Autodesk Inventor part; units mm, degrees
(part 2 of 2)
  line L765 (55.2108, -84.3874) -> (55.2873, -85.0207)
  line L766 (55.2873, -85.0207) -> (55.3337, -85.6628)
  line L767 (55.3337, -85.6628) -> (55.3494, -86.313)
  line L768 (75.3327, -73.346) -> (75.3327, -77.0507)
  line L769 (75.3327, -77.0507) -> (60.5124, -77.0507)
  line L770 (60.5124, -77.0507) -> (60.5124, -73.346)
  line L771 (60.5124, -73.346) -> (75.3327, -73.346)
  line L772 (60.513, -84.5139) -> (73.48, -84.5139)
  line L773 (73.48, -84.5139) -> (73.48, -88.1663)
  line L774 (73.48, -88.1663) -> (64.2178, -88.1663)
  line L775 (64.2178, -88.1663) -> (64.2178, -99.2813)
  line L776 (64.2178, -99.2813) -> (60.513, -99.2813)
  line L777 (60.513, -99.2813) -> (60.513, -84.5139)
  line L778 (79.5669, -73.346) -> (96.8562, -73.346)
  line L779 (96.8562, -73.346) -> (96.8562, -76.9851)
  line L780 (96.8562, -76.9851) -> (79.5669, -76.9851)
  line L781 (79.5669, -76.9851) -> (79.5669, -73.346)
  line L782 (86.3592, -99.2807) -> (86.3592, -79.0998)
  line L783 (86.3592, -79.0998) -> (90.064, -79.0998)
  line L784 (90.064, -79.0998) -> (90.064, -99.2813)
  line L785 (90.064, -99.2813) -> (86.3592, -99.2813)
  line L786 (86.3592, -99.2813) -> (86.3592, -99.2807)
  line L787 (108.9957, -95.7819) -> (108.9957, -99.5463)
  line L788 (108.9957, -99.5463) -> (108.5376, -99.5)
  line L789 (108.5376, -99.5) -> (108.0916, -99.4372)
  line L790 (108.0916, -99.4372) -> (107.6576, -99.3582)
  line L791 (107.6576, -99.3582) -> (107.2359, -99.2632)
  line L792 (107.2359, -99.2632) -> (106.8264, -99.1526)
  line L793 (106.8264, -99.1526) -> (106.4293, -99.0265)
  line L794 (106.4293, -99.0265) -> (106.0448, -98.8854)
  line L795 (106.0448, -98.8854) -> (105.6728, -98.7294)
  line L796 (105.6728, -98.7294) -> (105.3136, -98.5588)
  line L797 (105.3136, -98.5588) -> (104.9672, -98.374)
  line L798 (104.9672, -98.374) -> (104.6337, -98.1751)
  line L799 (104.6337, -98.1751) -> (104.3132, -97.9625)
  line L800 (104.3132, -97.9625) -> (104.0059, -97.7364)
  line L801 (104.0059, -97.7364) -> (103.7118, -97.4972)
  line L802 (103.7118, -97.4972) -> (103.431, -97.245)
  line L803 (103.431, -97.245) -> (103.1637, -96.9803)
  line L804 (103.1637, -96.9803) -> (102.9099, -96.7031)
  line L805 (102.9099, -96.7031) -> (102.6698, -96.4139)
  line L806 (102.6698, -96.4139) -> (102.4434, -96.1129)
  line L807 (102.4434, -96.1129) -> (102.2309, -95.8004)
  line L808 (102.2309, -95.8004) -> (102.0324, -95.4767)
  line L809 (102.0324, -95.4767) -> (101.8479, -95.1419)
  line L810 (101.8479, -95.1419) -> (101.6776, -94.7965)
  line L811 (101.6776, -94.7965) -> (101.5216, -94.4407)
  line L812 (101.5216, -94.4407) -> (101.38, -94.0748)
  line L813 (101.38, -94.0748) -> (101.2528, -93.6989)
  line L814 (101.2528, -93.6989) -> (101.1403, -93.3135)
  line L815 (101.1403, -93.3135) -> (101.0424, -92.9188)
  line L816 (101.0424, -92.9188) -> (100.9594, -92.5151)
  line L817 (100.9594, -92.5151) -> (100.8912, -92.1026)
  line L818 (100.8912, -92.1026) -> (100.8381, -91.6817)
  line L819 (100.8381, -91.6817) -> (100.8001, -91.2525)
  line L820 (100.8001, -91.2525) -> (104.5012, -90.6352)
  line L821 (104.5012, -90.6352) -> (104.5694, -91.1029)
  line L822 (104.5694, -91.1029) -> (104.6601, -91.56)
  line L823 (104.6601, -91.56) -> (104.7745, -92.0048)
  line L824 (104.7745, -92.0048) -> (104.9139, -92.4353)
  line L825 (104.9139, -92.4353) -> (105.0796, -92.8494)
  line L826 (105.0796, -92.8494) -> (105.2728, -93.2454)
  line L827 (105.2728, -93.2454) -> (105.4947, -93.6213)
  line L828 (105.4947, -93.6213) -> (105.7467, -93.9752)
  line L829 (105.7467, -93.9752) -> (106.0301, -94.3051)
  line L830 (106.0301, -94.3051) -> (106.3459, -94.6092)
  line L831 (106.3459, -94.6092) -> (106.6956, -94.8854)
  line L832 (106.6956, -94.8854) -> (107.0804, -95.1319)
  line L833 (107.0804, -95.1319) -> (107.2864, -95.2435)
  line L834 (107.2864, -95.2435) -> (107.5016, -95.3468)
  line L835 (107.5016, -95.3468) -> (107.7262, -95.4418)
  line L836 (107.7262, -95.4418) -> (107.9603, -95.5282)
  line L837 (107.9603, -95.5282) -> (108.2042, -95.6057)
  line L838 (108.2042, -95.6057) -> (108.4579, -95.674)
  line L839 (108.4579, -95.674) -> (108.7217, -95.7331)
  line L840 (108.7217, -95.7331) -> (108.9957, -95.7825)
  line L841 (108.9957, -95.7825) -> (108.9957, -95.7819)
  line L842 (108.9957, -73.0972) -> (108.9957, -76.8448)
  line L843 (108.9957, -76.8448) -> (108.7303, -76.8953)
  line L844 (108.7303, -76.8953) -> (108.4771, -76.9554)
  line L845 (108.4771, -76.9554) -> (108.2356, -77.0248)
  line L846 (108.2356, -77.0248) -> (108.0057, -77.1031)
  line L847 (108.0057, -77.1031) -> (107.787, -77.1901)
  line L848 (107.787, -77.1901) -> (107.5792, -77.2854)
  line L849 (107.5792, -77.2854) -> (107.3821, -77.3887)
  line L850 (107.3821, -77.3887) -> (107.1954, -77.4997)
  line L851 (107.1954, -77.4997) -> (107.0188, -77.6182)
  line L852 (107.0188, -77.6182) -> (106.8519, -77.7437)
  line L853 (106.8519, -77.7437) -> (106.5465, -78.0148)
  line L854 (106.5465, -78.0148) -> (106.2768, -78.3107)
  line L855 (106.2768, -78.3107) -> (106.0406, -78.6288)
  line L856 (106.0406, -78.6288) -> (105.8355, -78.9667)
  line L857 (105.8355, -78.9667) -> (105.6593, -79.3219)
  line L858 (105.6593, -79.3219) -> (105.5096, -79.692)
  line L859 (105.5096, -79.692) -> (105.3842, -80.0745)
  line L860 (105.3842, -80.0745) -> (105.2808, -80.467)
  line L861 (105.2808, -80.467) -> (105.1971, -80.8669)
  line L862 (105.1971, -80.8669) -> (105.1307, -81.2719)
  line L863 (105.1307, -81.2719) -> (105.0795, -81.6795)
  line L864 (105.0795, -81.6795) -> (101.3783, -81.0621)
  line L865 (101.3783, -81.0621) -> (101.4195, -80.6638)
  line L866 (101.4195, -80.6638) -> (101.4761, -80.272)
  line L867 (101.4761, -80.272) -> (101.5478, -79.8871)
  line L868 (101.5478, -79.8871) -> (101.6343, -79.5093)
  line L869 (101.6343, -79.5093) -> (101.7355, -79.139)
  line L870 (101.7355, -79.139) -> (101.8509, -78.7765)
  line L871 (101.8509, -78.7765) -> (101.9804, -78.422)
  line L872 (101.9804, -78.422) -> (102.1237, -78.076)
  line L873 (102.1237, -78.076) -> (102.2804, -77.7387)
  line L874 (102.2804, -77.7387) -> (102.4504, -77.4103)
  line L875 (102.4504, -77.4103) -> (102.6334, -77.0913)
  line L876 (102.6334, -77.0913) -> (102.829, -76.782)
  line L877 (102.829, -76.782) -> (103.0371, -76.4826)
  line L878 (103.0371, -76.4826) -> (103.2573, -76.1934)
  line L879 (103.2573, -76.1934) -> (103.4895, -75.9148)
  line L880 (103.4895, -75.9148) -> (103.7332, -75.6471)
  line L881 (103.7332, -75.6471) -> (103.9883, -75.3906)
  line L882 (103.9883, -75.3906) -> (104.2545, -75.1456)
  line L883 (104.2545, -75.1456) -> (104.5316, -74.9124)
  line L884 (104.5316, -74.9124) -> (104.8191, -74.6913)
  line L885 (104.8191, -74.6913) -> (105.117, -74.4827)
  line L886 (105.117, -74.4827) -> (105.4248, -74.2868)
  line L887 (105.4248, -74.2868) -> (105.7425, -74.1039)
  line L888 (105.7425, -74.1039) -> (106.0695, -73.9344)
  line L889 (106.0695, -73.9344) -> (106.4058, -73.7786)
  line L890 (106.4058, -73.7786) -> (106.751, -73.6367)
  line L891 (106.751, -73.6367) -> (107.1049, -73.5092)
  line L892 (107.1049, -73.5092) -> (107.4672, -73.3962)
  line L893 (107.4672, -73.3962) -> (107.8377, -73.2982)
  line L894 (107.8377, -73.2982) -> (108.216, -73.2153)
  line L895 (108.216, -73.2153) -> (108.6018, -73.148)
  line L896 (108.6018, -73.148) -> (108.9951, -73.0966)
  line L897 (108.9951, -73.0966) -> (108.9957, -73.0972)
  line L898 (119.306, -91.2525) -> (119.2993, -91.5962)
  line L899 (119.2993, -91.5962) -> (119.2793, -91.9424)
  line L900 (119.2793, -91.9424) -> (119.2455, -92.2901)
  line L901 (119.2455, -92.2901) -> (119.1978, -92.6387)
  line L902 (119.1978, -92.6387) -> (119.1358, -92.9874)
  line L903 (119.1358, -92.9874) -> (119.0594, -93.3353)
  line L904 (119.0594, -93.3353) -> (118.9681, -93.6817)
  line L905 (118.9681, -93.6817) -> (118.8619, -94.0258)
  line L906 (118.8619, -94.0258) -> (118.7403, -94.3667)
  line L907 (118.7403, -94.3667) -> (118.6032, -94.7039)
  line L908 (118.6032, -94.7039) -> (118.4503, -95.0363)
  line L909 (118.4503, -95.0363) -> (118.2812, -95.3633)
  line L910 (118.2812, -95.3633) -> (118.0958, -95.684)
  line L911 (118.0958, -95.684) -> (117.8938, -95.9977)
  line L912 (117.8938, -95.9977) -> (117.6749, -96.3036)
  line L913 (117.6749, -96.3036) -> (117.4388, -96.6009)
  line L914 (117.4388, -96.6009) -> (117.1853, -96.8889)
  line L915 (117.1853, -96.8889) -> (116.9141, -97.1666)
  line L916 (116.9141, -97.1666) -> (116.6249, -97.4334)
  line L917 (116.6249, -97.4334) -> (116.3175, -97.6884)
  line L918 (116.3175, -97.6884) -> (115.9917, -97.9309)
  line L919 (115.9917, -97.9309) -> (115.647, -98.16)
  line L920 (115.647, -98.16) -> (115.2834, -98.3751)
  line L921 (115.2834, -98.3751) -> (114.9004, -98.5752)
  line L922 (114.9004, -98.5752) -> (114.4979, -98.7597)
  line L923 (114.4979, -98.7597) -> (114.0756, -98.9277)
  line L924 (114.0756, -98.9277) -> (113.6331, -99.0784)
  line L925 (113.6331, -99.0784) -> (113.1704, -99.2111)
  line L926 (113.1704, -99.2111) -> (112.687, -99.325)
  line L927 (112.687, -99.325) -> (112.1827, -99.4192)
  line L928 (112.1827, -99.4192) -> (111.6572, -99.4931)
  line L929 (111.6572, -99.4931) -> (111.1104, -99.5457)
  line L930 (111.1104, -99.5457) -> (111.1104, -95.8234)
  line L931 (111.1104, -95.8234) -> (111.6337, -95.7501)
  line L932 (111.6337, -95.7501) -> (112.1273, -95.643)
  line L933 (112.1273, -95.643) -> (112.5907, -95.5038)
  line L934 (112.5907, -95.5038) -> (113.0232, -95.3344)
  line L935 (113.0232, -95.3344) -> (113.4244, -95.1363)
  line L936 (113.4244, -95.1363) -> (113.7936, -94.9114)
  line L937 (113.7936, -94.9114) -> (114.1303, -94.6612)
  line L938 (114.1303, -94.6612) -> (114.4339, -94.3877)
  line L939 (114.4339, -94.3877) -> (114.7039, -94.0924)
  line L940 (114.7039, -94.0924) -> (114.9397, -93.7771)
  line L941 (114.9397, -93.7771) -> (115.1408, -93.4436)
  line L942 (115.1408, -93.4436) -> (115.3065, -93.0934)
  line L943 (115.3065, -93.0934) -> (115.4364, -92.7284)
  line L944 (115.4364, -92.7284) -> (115.5299, -92.3503)
  line L945 (115.5299, -92.3503) -> (115.5864, -91.9608)
  line L946 (115.5864, -91.9608) -> (115.6054, -91.5615)
  line L947 (115.6054, -91.5615) -> (115.5845, -91.1111)
  line L948 (115.5845, -91.1111) -> (115.5227, -90.6978)
  line L949 (115.5227, -90.6978) -> (115.4769, -90.5047)
  line L950 (115.4769, -90.5047) -> (115.4214, -90.3202)
  line L951 (115.4214, -90.3202) -> (115.3564, -90.1443)
  line L952 (115.3564, -90.1443) -> (115.2819, -89.9768)
  line L953 (115.2819, -89.9768) -> (115.1982, -89.8174)
  line L954 (115.1982, -89.8174) -> (115.1055, -89.6659)
  line L955 (115.1055, -89.6659) -> (115.0038, -89.5222)
  line L956 (115.0038, -89.5222) -> (114.8935, -89.3861)
  line L957 (114.8935, -89.3861) -> (114.6473, -89.1357)
  line L958 (114.6473, -89.1357) -> (114.3682, -88.9133)
  line L959 (114.3682, -88.9133) -> (114.0575, -88.7174)
  line L960 (114.0575, -88.7174) -> (113.7166, -88.5462)
  line L961 (113.7166, -88.5462) -> (113.3467, -88.3985)
  line L962 (113.3467, -88.3985) -> (112.9493, -88.2725)
  line L963 (112.9493, -88.2725) -> (112.5256, -88.1667)
  line L964 (112.5256, -88.1667) -> (112.077, -88.0797)
  line L965 (112.077, -88.0797) -> (111.6048, -88.0098)
  line L966 (111.6048, -88.0098) -> (111.1104, -87.9555)
  line L967 (111.1104, -87.9555) -> (111.1104, -83.9201)
  line L968 (111.1104, -83.9201) -> (111.4723, -83.8432)
  line L969 (111.4723, -83.8432) -> (111.8318, -83.7523)
  line L970 (111.8318, -83.7523) -> (112.1858, -83.6464)
  line L971 (112.1858, -83.6464) -> (112.5315, -83.5245)
  line L972 (112.5315, -83.5245) -> (112.866, -83.3856)
  line L973 (112.866, -83.3856) -> (113.1866, -83.2287)
  line L974 (113.1866, -83.2287) -> (113.4902, -83.0527)
  line L975 (113.4902, -83.0527) -> (113.7741, -82.8567)
  line L976 (113.7741, -82.8567) -> (114.0353, -82.6396)
  line L977 (114.0353, -82.6396) -> (114.271, -82.4004)
  line L978 (114.271, -82.4004) -> (114.4783, -82.1382)
  line L979 (114.4783, -82.1382) -> (114.6544, -81.8519)
  line L980 (114.6544, -81.8519) -> (114.7963, -81.5404)
  line L981 (114.7963, -81.5404) -> (114.9012, -81.2029)
  line L982 (114.9012, -81.2029) -> (114.9389, -81.024)
  line L983 (114.9389, -81.024) -> (114.9663, -80.8382)
  line L984 (114.9663, -80.8382) -> (114.983, -80.6453)
  line L985 (114.983, -80.6453) -> (114.9886, -80.4453)
  line L986 (114.9886, -80.4453) -> (114.9742, -80.1536)
  line L987 (114.9742, -80.1536) -> (114.9307, -79.8588)
  line L988 (114.9307, -79.8588) -> (114.858, -79.5634)
  line L989 (114.858, -79.5634) -> (114.7556, -79.2699)
  line L990 (114.7556, -79.2699) -> (114.6233, -78.9808)
  line L991 (114.6233, -78.9808) -> (114.4608, -78.6986)
  line L992 (114.4608, -78.6986) -> (114.2678, -78.4258)
  line L993 (114.2678, -78.4258) -> (114.044, -78.1649)
  line L994 (114.044, -78.1649) -> (113.7891, -77.9184)
  line L995 (113.7891, -77.9184) -> (113.5029, -77.6888)
  line L996 (113.5029, -77.6888) -> (113.185, -77.4786)
  line L997 (113.185, -77.4786) -> (112.8351, -77.2902)
  line L998 (112.8351, -77.2902) -> (112.453, -77.1262)
  line L999 (112.453, -77.1262) -> (112.0384, -76.9891)
  line L1000 (112.0384, -76.9891) -> (111.5909, -76.8814)
  line L1001 (111.5909, -76.8814) -> (111.1104, -76.8056)
  line L1002 (111.1104, -76.8056) -> (111.1104, -73.0815)
  line L1003 (111.1104, -73.0815) -> (111.5953, -73.1345)
  line L1004 (111.5953, -73.1345) -> (112.0631, -73.2067)
  line L1005 (112.0631, -73.2067) -> (112.5138, -73.2973)
  line L1006 (112.5138, -73.2973) -> (112.9476, -73.4053)
  line L1007 (112.9476, -73.4053) -> (113.3645, -73.53)
  line L1008 (113.3645, -73.53) -> (113.7648, -73.6705)
  line L1009 (113.7648, -73.6705) -> (114.1484, -73.826)
  line L1010 (114.1484, -73.826) -> (114.5156, -73.9957)
  line L1011 (114.5156, -73.9957) -> (114.8665, -74.1786)
  line L1012 (114.8665, -74.1786) -> (115.201, -74.3741)
  line L1013 (115.201, -74.3741) -> (115.5195, -74.5812)
  line L1014 (115.5195, -74.5812) -> (115.822, -74.7991)
  line L1015 (115.822, -74.7991) -> (116.1085, -75.027)
  line L1016 (116.1085, -75.027) -> (116.3793, -75.264)
  line L1017 (116.3793, -75.264) -> (116.6345, -75.5093)
  line L1018 (116.6345, -75.5093) -> (116.8741, -75.762)
  line L1019 (116.8741, -75.762) -> (117.0982, -76.0214)
  line L1020 (117.0982, -76.0214) -> (117.3071, -76.2866)
  line L1021 (117.3071, -76.2866) -> (117.5008, -76.5567)
  line L1022 (117.5008, -76.5567) -> (117.6794, -76.8309)
  line L1023 (117.6794, -76.8309) -> (117.843, -77.1083)
  line L1024 (117.843, -77.1083) -> (117.9918, -77.3882)
  line L1025 (117.9918, -77.3882) -> (118.1259, -77.6697)
  line L1026 (118.1259, -77.6697) -> (118.2454, -77.952)
  line L1027 (118.2454, -77.952) -> (118.3503, -78.2342)
  line L1028 (118.3503, -78.2342) -> (118.4409, -78.5155)
  line L1029 (118.4409, -78.5155) -> (118.5173, -78.795)
  line L1030 (118.5173, -78.795) -> (118.5795, -79.0719)
  line L1031 (118.5795, -79.0719) -> (118.6276, -79.3454)
  line L1032 (118.6276, -79.3454) -> (118.6619, -79.6146)
  line L1033 (118.6619, -79.6146) -> (118.6824, -79.8788)
  line L1034 (118.6824, -79.8788) -> (118.6892, -80.137)
  line L1035 (118.6892, -80.137) -> (118.6783, -80.553)
  line L1036 (118.6783, -80.553) -> (118.6452, -80.9613)
  line L1037 (118.6452, -80.9613) -> (118.5895, -81.3614)
  line L1038 (118.5895, -81.3614) -> (118.5108, -81.7527)
  line L1039 (118.5108, -81.7527) -> (118.4086, -82.1347)
  line L1040 (118.4086, -82.1347) -> (118.2824, -82.5069)
  line L1041 (118.2824, -82.5069) -> (118.1319, -82.8689)
  line L1042 (118.1319, -82.8689) -> (117.9565, -83.22)
  line L1043 (117.9565, -83.22) -> (117.7558, -83.5599)
  line L1044 (117.7558, -83.5599) -> (117.5293, -83.8879)
  line L1045 (117.5293, -83.8879) -> (117.2767, -84.2036)
  line L1046 (117.2767, -84.2036) -> (116.9974, -84.5064)
  line L1047 (116.9974, -84.5064) -> (116.691, -84.796)
  line L1048 (116.691, -84.796) -> (116.3571, -85.0716)
  line L1049 (116.3571, -85.0716) -> (115.9952, -85.333)
  line L1050 (115.9952, -85.333) -> (115.6048, -85.5794)
  line L1051 (115.6048, -85.5794) -> (115.9641, -85.722)
  line L1052 (115.9641, -85.722) -> (116.3174, -85.9023)
  line L1053 (116.3174, -85.9023) -> (116.6623, -86.1183)
  line L1054 (116.6623, -86.1183) -> (116.9965, -86.3681)
  line L1055 (116.9965, -86.3681) -> (117.3175, -86.6495)
  line L1056 (117.3175, -86.6495) -> (117.6231, -86.9606)
  line L1057 (117.6231, -86.9606) -> (117.9108, -87.2992)
  line L1058 (117.9108, -87.2992) -> (118.1784, -87.6635)
  line L1059 (118.1784, -87.6635) -> (118.4233, -88.0512)
  line L1060 (118.4233, -88.0512) -> (118.6432, -88.4604)
  line L1061 (118.6432, -88.4604) -> (118.8359, -88.8891)
  line L1062 (118.8359, -88.8891) -> (118.9988, -89.3352)
  line L1063 (118.9988, -89.3352) -> (119.1296, -89.7967)
  line L1064 (119.1296, -89.7967) -> (119.226, -90.2716)
  line L1065 (119.226, -90.2716) -> (119.2856, -90.7577)
  line L1066 (119.2856, -90.7577) -> (119.306, -91.2531)
  line L1067 (119.306, -91.2531) -> (119.306, -91.2525)
  line L1068 (145.5665, -86.3136) -> (145.5526, -86.9824)
  line L1069 (145.5526, -86.9824) -> (145.5107, -87.6423)
  line L1070 (145.5107, -87.6423) -> (145.4413, -88.2924)
  line L1071 (145.4413, -88.2924) -> (145.3445, -88.9319)
  line L1072 (145.3445, -88.9319) -> (145.2204, -89.5601)
  line L1073 (145.2204, -89.5601) -> (145.0694, -90.1761)
  line L1074 (145.0694, -90.1761) -> (144.8915, -90.7791)
  line L1075 (144.8915, -90.7791) -> (144.687, -91.3683)
  line L1076 (144.687, -91.3683) -> (144.4562, -91.943)
  line L1077 (144.4562, -91.943) -> (144.1991, -92.5022)
  line L1078 (144.1991, -92.5022) -> (143.9161, -93.0452)
  line L1079 (143.9161, -93.0452) -> (143.6073, -93.5713)
  line L1080 (143.6073, -93.5713) -> (143.2729, -94.0795)
  line L1081 (143.2729, -94.0795) -> (142.9131, -94.5691)
  line L1082 (142.9131, -94.5691) -> (142.5282, -95.0393)
  line L1083 (142.5282, -95.0393) -> (142.1183, -95.4892)
  line L1084 (142.1183, -95.4892) -> (141.6836, -95.9182)
  line L1085 (141.6836, -95.9182) -> (141.2243, -96.3253)
  line L1086 (141.2243, -96.3253) -> (140.7408, -96.7097)
  line L1087 (140.7408, -96.7097) -> (140.233, -97.0707)
  line L1088 (140.233, -97.0707) -> (139.7013, -97.4074)
  line L1089 (139.7013, -97.4074) -> (139.1459, -97.7191)
  line L1090 (139.1459, -97.7191) -> (138.567, -98.005)
  line L1091 (138.567, -98.005) -> (137.9647, -98.2641)
  line L1092 (137.9647, -98.2641) -> (137.3393, -98.4958)
  line L1093 (137.3393, -98.4958) -> (136.6909, -98.6992)
  line L1094 (136.6909, -98.6992) -> (136.0198, -98.8735)
  line L1095 (136.0198, -98.8735) -> (135.3263, -99.018)
  line L1096 (135.3263, -99.018) -> (134.6104, -99.1317)
  line L1097 (134.6104, -99.1317) -> (133.8724, -99.2139)
  line L1098 (133.8724, -99.2139) -> (133.1124, -99.2639)
  line L1099 (133.1124, -99.2639) -> (132.3308, -99.2807)
  line L1100 (132.3308, -99.2807) -> (124.5737, -99.2807)
  line L1101 (124.5737, -99.2807) -> (124.5737, -84.5139)
  line L1102 (124.5737, -84.5139) -> (128.2857, -84.5139)
  line L1103 (128.2857, -84.5139) -> (128.2857, -95.5759)
  line L1104 (128.2857, -95.5759) -> (133.2945, -95.5759)
  line L1105 (133.2945, -95.5759) -> (133.764, -95.5639)
  line L1106 (133.764, -95.5639) -> (134.2241, -95.5283)
  line L1107 (134.2241, -95.5283) -> (134.6744, -95.4696)
  line L1108 (134.6744, -95.4696) -> (135.1146, -95.3884)
  line L1109 (135.1146, -95.3884) -> (135.5443, -95.2853)
  line L1110 (135.5443, -95.2853) -> (135.9632, -95.1609)
  line L1111 (135.9632, -95.1609) -> (136.3708, -95.0157)
  line L1112 (136.3708, -95.0157) -> (136.7668, -94.8504)
  line L1113 (136.7668, -94.8504) -> (137.151, -94.6654)
  line L1114 (137.151, -94.6654) -> (137.5228, -94.4614)
  line L1115 (137.5228, -94.4614) -> (137.882, -94.2389)
  line L1116 (137.882, -94.2389) -> (138.2281, -93.9985)
  line L1117 (138.2281, -93.9985) -> (138.5609, -93.7407)
  line L1118 (138.5609, -93.7407) -> (138.88, -93.4662)
  line L1119 (138.88, -93.4662) -> (139.1849, -93.1756)
  line L1120 (139.1849, -93.1756) -> (139.4754, -92.8693)
  line L1121 (139.4754, -92.8693) -> (139.7511, -92.548)
  line L1122 (139.7511, -92.548) -> (140.0116, -92.2122)
  line L1123 (140.0116, -92.2122) -> (140.2566, -91.8625)
  line L1124 (140.2566, -91.8625) -> (140.4856, -91.4995)
  line L1125 (140.4856, -91.4995) -> (140.6985, -91.1238)
  line L1126 (140.6985, -91.1238) -> (140.8947, -90.7358)
  line L1127 (140.8947, -90.7358) -> (141.0739, -90.3363)
  line L1128 (141.0739, -90.3363) -> (141.2358, -89.9258)
  line L1129 (141.2358, -89.9258) -> (141.38, -89.5048)
  line L1130 (141.38, -89.5048) -> (141.5061, -89.0739)
  line L1131 (141.5061, -89.0739) -> (141.6138, -88.6337)
  line L1132 (141.6138, -88.6337) -> (141.7028, -88.1847)
  line L1133 (141.7028, -88.1847) -> (141.7726, -87.7276)
  line L1134 (141.7726, -87.7276) -> (141.8229, -87.2629)
  line L1135 (141.8229, -87.2629) -> (141.8533, -86.7912)
  line L1136 (141.8533, -86.7912) -> (141.8635, -86.313)
  line L1137 (141.8635, -86.313) -> (141.8533, -85.8348)
  line L1138 (141.8533, -85.8348) -> (141.8229, -85.3631)
  line L1139 (141.8229, -85.3631) -> (141.7726, -84.8984)
  line L1140 (141.7726, -84.8984) -> (141.7028, -84.4413)
  line L1141 (141.7028, -84.4413) -> (141.6138, -83.9924)
  line L1142 (141.6138, -83.9924) -> (141.5061, -83.5522)
  line L1143 (141.5061, -83.5522) -> (141.38, -83.1213)
  line L1144 (141.38, -83.1213) -> (141.2358, -82.7003)
  line L1145 (141.2358, -82.7003) -> (141.0739, -82.2897)
  line L1146 (141.0739, -82.2897) -> (140.8947, -81.8902)
  line L1147 (140.8947, -81.8902) -> (140.6985, -81.5023)
  line L1148 (140.6985, -81.5023) -> (140.4856, -81.1265)
  line L1149 (140.4856, -81.1265) -> (140.2566, -80.7635)
  line L1150 (140.2566, -80.7635) -> (140.0116, -80.4139)
  line L1151 (140.0116, -80.4139) -> (139.7511, -80.0781)
  line L1152 (139.7511, -80.0781) -> (139.4754, -79.7568)
  line L1153 (139.4754, -79.7568) -> (139.1849, -79.4505)
  line L1154 (139.1849, -79.4505) -> (138.88, -79.1598)
  line L1155 (138.88, -79.1598) -> (138.5609, -78.8853)
  line L1156 (138.5609, -78.8853) -> (138.2281, -78.6276)
  line L1157 (138.2281, -78.6276) -> (137.882, -78.3872)
  line L1158 (137.882, -78.3872) -> (137.5228, -78.1647)
  line L1159 (137.5228, -78.1647) -> (137.151, -77.9606)
  line L1160 (137.151, -77.9606) -> (136.7668, -77.7757)
  line L1161 (136.7668, -77.7757) -> (136.3708, -77.6103)
  line L1162 (136.3708, -77.6103) -> (135.9632, -77.4651)
  line L1163 (135.9632, -77.4651) -> (135.5443, -77.3407)
  line L1164 (135.5443, -77.3407) -> (135.1146, -77.2376)
  line L1165 (135.1146, -77.2376) -> (134.6744, -77.1565)
  line L1166 (134.6744, -77.1565) -> (134.2241, -77.0978)
  line L1167 (134.2241, -77.0978) -> (133.764, -77.0621)
  line L1168 (133.764, -77.0621) -> (133.2945, -77.0501)
  line L1169 (133.2945, -77.0501) -> (124.5737, -77.0501)
  line L1170 (124.5737, -77.0501) -> (124.5737, -73.3454)
  line L1171 (124.5737, -73.3454) -> (132.3308, -73.3454)
  line L1172 (132.3308, -73.3454) -> (133.1294, -73.3622)
  line L1173 (133.1294, -73.3622) -> (133.9041, -73.4121)
  line L1174 (133.9041, -73.4121) -> (134.6549, -73.4943)
  line L1175 (134.6549, -73.4943) -> (135.3817, -73.6081)
  line L1176 (135.3817, -73.6081) -> (136.0843, -73.7525)
  line L1177 (136.0843, -73.7525) -> (136.7626, -73.9268)
  line L1178 (136.7626, -73.9268) -> (137.4167, -74.1302)
  line L1179 (137.4167, -74.1302) -> (138.0462, -74.3619)
  line L1180 (138.0462, -74.3619) -> (138.6513, -74.6211)
  line L1181 (138.6513, -74.6211) -> (139.2317, -74.9069)
  line L1182 (139.2317, -74.9069) -> (139.7874, -75.2186)
  line L1183 (139.7874, -75.2186) -> (140.3182, -75.5553)
  line L1184 (140.3182, -75.5553) -> (140.8241, -75.9163)
  line L1185 (140.8241, -75.9163) -> (141.305, -76.3008)
  line L1186 (141.305, -76.3008) -> (141.7607, -76.7079)
  line L1187 (141.7607, -76.7079) -> (142.1912, -77.1368)
  line L1188 (142.1912, -77.1368) -> (142.5964, -77.5868)
  line L1189 (142.5964, -77.5868) -> (142.9761, -78.0569)
  line L1190 (142.9761, -78.0569) -> (143.3303, -78.5465)
  line L1191 (143.3303, -78.5465) -> (143.6589, -79.0548)
  line L1192 (143.6589, -79.0548) -> (143.9617, -79.5808)
  line L1193 (143.9617, -79.5808) -> (144.2388, -80.1238)
  line L1194 (144.2388, -80.1238) -> (144.4898, -80.6831)
  line L1195 (144.4898, -80.6831) -> (144.7149, -81.2577)
  line L1196 (144.7149, -81.2577) -> (144.9138, -81.8469)
  line L1197 (144.9138, -81.8469) -> (145.0866, -82.45)
  line L1198 (145.0866, -82.45) -> (145.2329, -83.0659)
  line L1199 (145.2329, -83.0659) -> (145.3529, -83.6941)
  line L1200 (145.3529, -83.6941) -> (145.4463, -84.3336)
  line L1201 (145.4463, -84.3336) -> (145.5132, -84.9837)
  line L1202 (145.5132, -84.9837) -> (145.5533, -85.6436)
  line L1203 (145.5533, -85.6436) -> (145.5665, -86.3124)
  line L1204 (145.5665, -86.3124) -> (145.5665, -86.3136)
  line L1205 (-67.9151, -73.346) -> (-53.096, -73.346)
  line L1206 (-53.096, -73.346) -> (-53.096, -77.0507)
  line L1207 (-53.096, -77.0507) -> (-67.9151, -77.0507)
  line L1208 (-67.9151, -77.0507) -> (-67.9151, -73.346)
  line L1209 (-67.9151, -84.5145) -> (-54.9475, -84.5145)
  line L1210 (-54.9475, -84.5145) -> (-54.9475, -88.1669)
  line L1211 (-54.9475, -88.1669) -> (-64.2013, -88.1669)
  line L1212 (-64.2013, -88.1669) -> (-64.2013, -95.5765)
  line L1213 (-64.2013, -95.5765) -> (-53.0942, -95.5765)
  line L1214 (-53.0942, -95.5765) -> (-53.0942, -99.2813)
  line L1215 (-53.0942, -99.2813) -> (-67.9151, -99.2813)
  line L1216 (-67.9151, -99.2813) -> (-67.9151, -84.5145)
  line L1217 (-114.2777, -90.8436) -> (-114.3482, -90.2478)
  line L1218 (-114.3482, -90.2478) -> (-114.4336, -89.6547)
  line L1219 (-114.4336, -89.6547) -> (-114.5338, -89.0648)
  line L1220 (-114.5338, -89.0648) -> (-114.6487, -88.4782)
  line L1221 (-114.6487, -88.4782) -> (-114.7781, -87.8952)
  line L1222 (-114.7781, -87.8952) -> (-114.9219, -87.3161)
  line L1223 (-114.9219, -87.3161) -> (-115.0798, -86.7412)
  line L1224 (-115.0798, -86.7412) -> (-115.2519, -86.1706)
  line L1225 (-115.2519, -86.1706) -> (-115.4378, -85.6048)
  line L1226 (-115.4378, -85.6048) -> (-115.6376, -85.0439)
  line L1227 (-115.6376, -85.0439) -> (-115.851, -84.4883)
  line L1228 (-115.851, -84.4883) -> (-116.0778, -83.9382)
  line L1229 (-116.0778, -83.9382) -> (-116.3181, -83.3938)
  line L1230 (-116.3181, -83.3938) -> (-116.5715, -82.8555)
  line L1231 (-116.5715, -82.8555) -> (-116.838, -82.3235)
  line L1232 (-116.838, -82.3235) -> (-117.1173, -81.7981)
  line L1233 (-117.1173, -81.7981) -> (-117.4095, -81.2795)
  line L1234 (-117.4095, -81.2795) -> (-117.7143, -80.768)
  line L1235 (-117.7143, -80.768) -> (-118.0315, -80.264)
  line L1236 (-118.0315, -80.264) -> (-118.3611, -79.7676)
  line L1237 (-118.3611, -79.7676) -> (-118.7028, -79.2791)
  line L1238 (-118.7028, -79.2791) -> (-119.0566, -78.7988)
  line L1239 (-119.0566, -78.7988) -> (-119.4223, -78.327)
  line L1240 (-119.4223, -78.327) -> (-119.7997, -77.864)
  line L1241 (-119.7997, -77.864) -> (-120.1887, -77.4099)
  line L1242 (-120.1887, -77.4099) -> (-120.5892, -76.9652)
  line L1243 (-120.5892, -76.9652) -> (-121.0009, -76.53)
  line L1244 (-121.0009, -76.53) -> (-121.4239, -76.1046)
  line L1245 (-121.4239, -76.1046) -> (-121.8578, -75.6893)
  line L1246 (-121.8578, -75.6893) -> (-122.3027, -75.2843)
  line L1247 (-122.3027, -75.2843) -> (-122.7582, -74.89)
  line L1248 (-122.7582, -74.89) -> (-123.2244, -74.5066)
  line L1249 (-123.2244, -74.5066) -> (-123.3195, -74.4295)
  line L1250 (-123.3195, -74.4295) -> (-123.3665, -74.3916)
  line L1251 (-123.3665, -74.3916) -> (-124.0523, -73.8698)
  line L1252 (-124.0523, -73.8698) -> (-124.7532, -73.3742)
  line L1253 (-124.7532, -73.3742) -> (-125.4685, -72.9052)
  line L1254 (-125.4685, -72.9052) -> (-126.1977, -72.4629)
  line L1255 (-126.1977, -72.4629) -> (-126.9401, -72.0475)
  line L1256 (-126.9401, -72.0475) -> (-127.6952, -71.6594)
  line L1257 (-127.6952, -71.6594) -> (-128.4622, -71.2988)
  line L1258 (-128.4622, -71.2988) -> (-129.2407, -70.9659)
  line L1259 (-129.2407, -70.9659) -> (-130.0299, -70.6609)
  line L1260 (-130.0299, -70.6609) -> (-130.8292, -70.3841)
  line L1261 (-130.8292, -70.3841) -> (-131.6381, -70.1357)
  line L1262 (-131.6381, -70.1357) -> (-132.4559, -69.916)
  line L1263 (-132.4559, -69.916) -> (-133.2821, -69.7251)
  line L1264 (-133.2821, -69.7251) -> (-134.1159, -69.5635)
  line L1265 (-134.1159, -69.5635) -> (-134.9568, -69.4312)
  line L1266 (-134.9568, -69.4312) -> (-135.8041, -69.3286)
  line L1267 (-135.8041, -69.3286) -> (-135.1476, -68.8902)
  line L1268 (-135.1476, -68.8902) -> (-134.4753, -68.4777)
  line L1269 (-134.4753, -68.4777) -> (-133.788, -68.0914)
  line L1270 (-133.788, -68.0914) -> (-133.0869, -67.7316)
  line L1271 (-133.0869, -67.7316) -> (-132.373, -67.3986)
  line L1272 (-132.373, -67.3986) -> (-131.6473, -67.0928)
  line L1273 (-131.6473, -67.0928) -> (-130.9107, -66.8146)
  line L1274 (-130.9107, -66.8146) -> (-130.1644, -66.5642)
  line L1275 (-130.1644, -66.5642) -> (-129.4092, -66.342)
  line L1276 (-129.4092, -66.342) -> (-128.6463, -66.1484)
  line L1277 (-128.6463, -66.1484) -> (-127.8766, -65.9836)
  line L1278 (-127.8766, -65.9836) -> (-127.1012, -65.848)
  line L1279 (-127.1012, -65.848) -> (-126.321, -65.742)
  line L1280 (-126.321, -65.742) -> (-125.5371, -65.6658)
  line L1281 (-125.5371, -65.6658) -> (-124.7505, -65.6199)
  line L1282 (-124.7505, -65.6199) -> (-123.9622, -65.6045)
  line L1283 (-123.9622, -65.6045) -> (-123.4315, -65.6111)
  line L1284 (-123.4315, -65.6111) -> (-122.9031, -65.6308)
  line L1285 (-122.9031, -65.6308) -> (-122.3773, -65.6636)
  line L1286 (-122.3773, -65.6636) -> (-121.8542, -65.7094)
  line L1287 (-121.8542, -65.7094) -> (-121.3341, -65.7681)
  line L1288 (-121.3341, -65.7681) -> (-120.817, -65.8396)
  line L1289 (-120.817, -65.8396) -> (-120.3032, -65.9239)
  line L1290 (-120.3032, -65.9239) -> (-119.7928, -66.0208)
  line L1291 (-119.7928, -66.0208) -> (-119.2861, -66.1304)
  line L1292 (-119.2861, -66.1304) -> (-118.7832, -66.2525)
  line L1293 (-118.7832, -66.2525) -> (-118.2842, -66.387)
  line L1294 (-118.2842, -66.387) -> (-117.7895, -66.534)
  line L1295 (-117.7895, -66.534) -> (-117.299, -66.6932)
  line L1296 (-117.299, -66.6932) -> (-116.8131, -66.8646)
  line L1297 (-116.8131, -66.8646) -> (-116.3319, -67.0482)
  line L1298 (-116.3319, -67.0482) -> (-115.8555, -67.2439)
  line L1299 (-115.8555, -67.2439) -> (-115.3842, -67.4516)
  line L1300 (-115.3842, -67.4516) -> (-114.9182, -67.6712)
  line L1301 (-114.9182, -67.6712) -> (-114.4575, -67.9026)
  line L1302 (-114.4575, -67.9026) -> (-114.0025, -68.1458)
  line L1303 (-114.0025, -68.1458) -> (-113.5532, -68.4007)
  line L1304 (-113.5532, -68.4007) -> (-113.1098, -68.6672)
  line L1305 (-113.1098, -68.6672) -> (-112.6726, -68.9453)
  line L1306 (-112.6726, -68.9453) -> (-112.2417, -69.2348)
  line L1307 (-112.2417, -69.2348) -> (-111.8173, -69.5357)
  line L1308 (-111.8173, -69.5357) -> (-111.3996, -69.8479)
  line L1309 (-111.3996, -69.8479) -> (-110.9887, -70.1714)
  line L1310 (-110.9887, -70.1714) -> (-110.5848, -70.506)
  line L1311 (-110.5848, -70.506) -> (-110.1881, -70.8517)
  line L1312 (-110.1881, -70.8517) -> (-109.7988, -71.2085)
  line L1313 (-109.7988, -71.2085) -> (-109.4171, -71.5761)
  line L1314 (-109.4171, -71.5761) -> (-109.043, -71.9546)
  line L1315 (-109.043, -71.9546) -> (-108.8943, -72.1088)
  line L1316 (-108.8943, -72.1088) -> (-108.8708, -72.1335)
  line L1317 (-108.8708, -72.1335) -> (-108.444, -72.6003)
  line L1318 (-108.444, -72.6003) -> (-108.0321, -73.0793)
  line L1319 (-108.0321, -73.0793) -> (-107.6353, -73.5703)
  line L1320 (-107.6353, -73.5703) -> (-107.2539, -74.0727)
  line L1321 (-107.2539, -74.0727) -> (-106.8881, -74.586)
  line L1322 (-106.8881, -74.586) -> (-106.5382, -75.1097)
  line L1323 (-106.5382, -75.1097) -> (-106.2044, -75.6435)
  line L1324 (-106.2044, -75.6435) -> (-105.8871, -76.1868)
  line L1325 (-105.8871, -76.1868) -> (-105.5865, -76.7392)
  line L1326 (-105.5865, -76.7392) -> (-105.3027, -77.3002)
  line L1327 (-105.3027, -77.3002) -> (-105.0362, -77.8693)
  line L1328 (-105.0362, -77.8693) -> (-104.7871, -78.4461)
  line L1329 (-104.7871, -78.4461) -> (-104.5557, -79.0301)
  line L1330 (-104.5557, -79.0301) -> (-104.3423, -79.6208)
  line L1331 (-104.3423, -79.6208) -> (-104.1471, -80.2178)
  line L1332 (-104.1471, -80.2178) -> (-103.9704, -80.8206)
  line L1333 (-103.9704, -80.8206) -> (-104.4077, -81.6286)
  line L1334 (-104.4077, -81.6286) -> (-104.8769, -82.4166)
  line L1335 (-104.8769, -82.4166) -> (-105.3771, -83.1837)
  line L1336 (-105.3771, -83.1837) -> (-105.9074, -83.929)
  line L1337 (-105.9074, -83.929) -> (-106.4669, -84.6515)
  line L1338 (-106.4669, -84.6515) -> (-107.0545, -85.3504)
  line L1339 (-107.0545, -85.3504) -> (-107.6694, -86.0249)
  line L1340 (-107.6694, -86.0249) -> (-108.3106, -86.6739)
  line L1341 (-108.3106, -86.6739) -> (-108.9773, -87.2966)
  line L1342 (-108.9773, -87.2966) -> (-109.6684, -87.8921)
  line L1343 (-109.6684, -87.8921) -> (-110.3831, -88.4595)
  line L1344 (-110.3831, -88.4595) -> (-111.1204, -88.9979)
  line L1345 (-111.1204, -88.9979) -> (-111.8794, -89.5064)
  line L1346 (-111.8794, -89.5064) -> (-112.6591, -89.9841)
  line L1347 (-112.6591, -89.9841) -> (-113.4587, -90.4301)
  line L1348 (-113.4587, -90.4301) -> (-114.2771, -90.8436)
  line L1349 (-114.2771, -90.8436) -> (-114.2777, -90.8436)
  line L1350 (-129.8491, -106.2229) -> (-130.6639, -105.9631)
  line L1351 (-130.6639, -105.9631) -> (-131.4623, -105.672)
  line L1352 (-131.4623, -105.672) -> (-132.2436, -105.3503)
  line L1353 (-132.2436, -105.3503) -> (-133.0071, -104.999)
  line L1354 (-133.0071, -104.999) -> (-133.7524, -104.6188)
  line L1355 (-133.7524, -104.6188) -> (-134.4787, -104.2104)
  line L1356 (-134.4787, -104.2104) -> (-135.1855, -103.7747)
  line L1357 (-135.1855, -103.7747) -> (-135.8722, -103.3125)
  line L1358 (-135.8722, -103.3125) -> (-136.538, -102.8246)
  line L1359 (-136.538, -102.8246) -> (-137.1825, -102.3117)
  line L1360 (-137.1825, -102.3117) -> (-137.8049, -101.7748)
  line L1361 (-137.8049, -101.7748) -> (-138.4047, -101.2145)
  line L1362 (-138.4047, -101.2145) -> (-138.9813, -100.6316)
  line L1363 (-138.9813, -100.6316) -> (-139.534, -100.0271)
  line L1364 (-139.534, -100.0271) -> (-140.0622, -99.4016)
  line L1365 (-140.0622, -99.4016) -> (-140.5654, -98.7559)
  line L1366 (-140.5654, -98.7559) -> (-141.0428, -98.091)
  line L1367 (-141.0428, -98.091) -> (-141.4939, -97.4075)
  line L1368 (-141.4939, -97.4075) -> (-141.918, -96.7062)
  line L1369 (-141.918, -96.7062) -> (-142.3146, -95.988)
  line L1370 (-142.3146, -95.988) -> (-142.683, -95.2537)
  line L1371 (-142.683, -95.2537) -> (-143.0226, -94.504)
  line L1372 (-143.0226, -94.504) -> (-143.3328, -93.7398)
  line L1373 (-143.3328, -93.7398) -> (-143.613, -92.9618)
  line L1374 (-143.613, -92.9618) -> (-143.8625, -92.1709)
  line L1375 (-143.8625, -92.1709) -> (-144.0807, -91.3678)
  line L1376 (-144.0807, -91.3678) -> (-144.2671, -90.5534)
  line L1377 (-144.2671, -90.5534) -> (-144.4209, -89.7284)
  line L1378 (-144.4209, -89.7284) -> (-144.5417, -88.8937)
  line L1379 (-144.5417, -88.8937) -> (-144.6287, -88.05)
  line L1380 (-144.6287, -88.05) -> (-144.6813, -87.1981)
  line L1381 (-144.6813, -87.1981) -> (-144.699, -86.3389)
  line L1382 (-144.699, -86.3389) -> (-144.6928, -85.8325)
  line L1383 (-144.6928, -85.8325) -> (-144.6743, -85.3263)
  line L1384 (-144.6743, -85.3263) -> (-144.6435, -84.8207)
  line L1385 (-144.6435, -84.8207) -> (-144.6005, -84.3162)
  line L1386 (-144.6005, -84.3162) -> (-144.5452, -83.8133)
  line L1387 (-144.5452, -83.8133) -> (-144.4777, -83.3123)
  line L1388 (-144.4777, -83.3123) -> (-144.3981, -82.8137)
  line L1389 (-144.3981, -82.8137) -> (-144.3063, -82.3179)
  line L1390 (-144.3063, -82.3179) -> (-144.2509, -82.0397)
  line L1391 (-144.2509, -82.0397) -> (-144.0919, -81.3488)
  line L1392 (-144.0919, -81.3488) -> (-143.9095, -80.6652)
  line L1393 (-143.9095, -80.6652) -> (-143.7041, -79.9892)
  line L1394 (-143.7041, -79.9892) -> (-143.4759, -79.3215)
  line L1395 (-143.4759, -79.3215) -> (-143.2253, -78.6625)
  line L1396 (-143.2253, -78.6625) -> (-142.9524, -78.0128)
  line L1397 (-142.9524, -78.0128) -> (-142.6576, -77.3729)
  line L1398 (-142.6576, -77.3729) -> (-142.3412, -76.7434)
  line L1399 (-142.3412, -76.7434) -> (-142.0034, -76.1248)
  line L1400 (-142.0034, -76.1248) -> (-141.6446, -75.5177)
  line L1401 (-141.6446, -75.5177) -> (-141.265, -74.9226)
  line L1402 (-141.265, -74.9226) -> (-140.8649, -74.34)
  line L1403 (-140.8649, -74.34) -> (-140.4445, -73.7704)
  line L1404 (-140.4445, -73.7704) -> (-140.0043, -73.2145)
  line L1405 (-140.0043, -73.2145) -> (-139.5443, -72.6727)
  line L1406 (-139.5443, -72.6727) -> (-139.065, -72.1456)
  line L1407 (-139.065, -72.1456) -> (-138.9006, -71.9733)
  line L1408 (-138.9006, -71.9733) -> (-138.3603, -71.4324)
  line L1409 (-138.3603, -71.4324) -> (-137.8068, -70.9168)
  line L1410 (-137.8068, -70.9168) -> (-136.9557, -70.9519)
  line L1411 (-136.9557, -70.9519) -> (-136.1103, -71.0184)
  line L1412 (-136.1103, -71.0184) -> (-135.2711, -71.1163)
  line L1413 (-135.2711, -71.1163) -> (-134.4387, -71.2452)
  line L1414 (-134.4387, -71.2452) -> (-133.614, -71.4049)
  line L1415 (-133.614, -71.4049) -> (-132.7974, -71.5953)
  line L1416 (-132.7974, -71.5953) -> (-131.9896, -71.8161)
  line L1417 (-131.9896, -71.8161) -> (-131.1914, -72.0671)
  line L1418 (-131.1914, -72.0671) -> (-130.4033, -72.3481)
  line L1419 (-130.4033, -72.3481) -> (-129.6259, -72.6588)
  line L1420 (-129.6259, -72.6588) -> (-128.86, -72.999)
  line L1421 (-128.86, -72.999) -> (-128.1062, -73.3686)
  line L1422 (-128.1062, -73.3686) -> (-127.3651, -73.7672)
  line L1423 (-127.3651, -73.7672) -> (-126.6374, -74.1947)
  line L1424 (-126.6374, -74.1947) -> (-125.9237, -74.6508)
  line L1425 (-125.9237, -74.6508) -> (-125.2246, -75.1354)
  line L1426 (-125.2246, -75.1354) -> (-125.6802, -75.5423)
  line L1427 (-125.6802, -75.5423) -> (-126.1246, -75.9599)
  line L1428 (-126.1246, -75.9599) -> (-126.5575, -76.3878)
  line L1429 (-126.5575, -76.3878) -> (-126.9788, -76.8257)
  line L1430 (-126.9788, -76.8257) -> (-127.3884, -77.2734)
  line L1431 (-127.3884, -77.2734) -> (-127.7862, -77.7306)
  line L1432 (-127.7862, -77.7306) -> (-128.172, -78.197)
  line L1433 (-128.172, -78.197) -> (-128.5456, -78.6724)
  line L1434 (-128.5456, -78.6724) -> (-128.907, -79.1564)
  line L1435 (-128.907, -79.1564) -> (-129.256, -79.6488)
  line L1436 (-129.256, -79.6488) -> (-129.5925, -80.1494)
  line L1437 (-129.5925, -80.1494) -> (-129.9162, -80.6577)
  line L1438 (-129.9162, -80.6577) -> (-130.2272, -81.1736)
  line L1439 (-130.2272, -81.1736) -> (-130.5252, -81.6968)
  line L1440 (-130.5252, -81.6968) -> (-130.81, -82.2269)
  line L1441 (-130.81, -82.2269) -> (-131.0817, -82.7638)
  line L1442 (-131.0817, -82.7638) -> (-131.34, -83.3071)
  line L1443 (-131.34, -83.3071) -> (-131.5847, -83.8565)
  line L1444 (-131.5847, -83.8565) -> (-131.8158, -84.4119)
  line L1445 (-131.8158, -84.4119) -> (-132.0331, -84.9728)
  line L1446 (-132.0331, -84.9728) -> (-132.2365, -85.539)
  line L1447 (-132.2365, -85.539) -> (-132.4258, -86.1103)
  line L1448 (-132.4258, -86.1103) -> (-132.6009, -86.6864)
  line L1449 (-132.6009, -86.6864) -> (-132.7616, -87.2669)
  line L1450 (-132.7616, -87.2669) -> (-132.9078, -87.8516)
  line L1451 (-132.9078, -87.8516) -> (-133.0395, -88.4403)
  line L1452 (-133.0395, -88.4403) -> (-133.1563, -89.0326)
  line L1453 (-133.1563, -89.0326) -> (-133.2583, -89.6283)
  line L1454 (-133.2583, -89.6283) -> (-133.3452, -90.2271)
  line L1455 (-133.3452, -90.2271) -> (-133.4169, -90.8287)
  line L1456 (-133.4169, -90.8287) -> (-133.4733, -91.4328)
  line L1457 (-133.4733, -91.4328) -> (-133.5142, -92.0392)
  line L1458 (-133.5142, -92.0392) -> (-133.5238, -92.25)
  line L1459 (-133.5238, -92.25) -> (-133.5444, -92.8069)
  line L1460 (-133.5444, -92.8069) -> (-133.5515, -93.3775)
  line L1461 (-133.5515, -93.3775) -> (-133.5367, -94.2247)
  line L1462 (-133.5367, -94.2247) -> (-133.4925, -95.0687)
  line L1463 (-133.4925, -95.0687) -> (-133.4191, -95.9087)
  line L1464 (-133.4191, -95.9087) -> (-133.3166, -96.744)
  line L1465 (-133.3166, -96.744) -> (-133.1853, -97.5739)
  line L1466 (-133.1853, -97.5739) -> (-133.0254, -98.3977)
  line L1467 (-133.0254, -98.3977) -> (-132.8371, -99.2147)
  line L1468 (-132.8371, -99.2147) -> (-132.6205, -100.0242)
  line L1469 (-132.6205, -100.0242) -> (-132.3759, -100.8256)
  line L1470 (-132.3759, -100.8256) -> (-132.1035, -101.618)
  line L1471 (-132.1035, -101.618) -> (-131.8035, -102.4009)
  line L1472 (-131.8035, -102.4009) -> (-131.476, -103.1735)
  line L1473 (-131.476, -103.1735) -> (-131.1214, -103.9351)
  line L1474 (-131.1214, -103.9351) -> (-130.7397, -104.685)
  line L1475 (-130.7397, -104.685) -> (-130.3312, -105.4225)
  line L1476 (-130.3312, -105.4225) -> (-129.8961, -106.147)
  line L1477 (-129.8961, -106.147) -> (-129.8491, -106.2223)
  line L1478 (-129.8491, -106.2223) -> (-129.8491, -106.2229)
  line L1479 (-123.9622, -107.0757) -> (-124.8218, -107.0579)
  line L1480 (-124.8218, -107.0579) -> (-125.6803, -107.0047)
  line L1481 (-125.6803, -107.0047) -> (-126.5349, -106.9164)
  line L1482 (-126.5349, -106.9164) -> (-127.3827, -106.7933)
  line L1483 (-127.3827, -106.7933) -> (-127.8061, -106.2066)
  line L1484 (-127.8061, -106.2066) -> (-128.2097, -105.6073)
  line L1485 (-128.2097, -105.6073) -> (-128.3482, -105.3929)
  line L1486 (-128.3482, -105.3929) -> (-128.7619, -104.7161)
  line L1487 (-128.7619, -104.7161) -> (-129.1504, -104.0268)
  line L1488 (-129.1504, -104.0268) -> (-129.5135, -103.3257)
  line L1489 (-129.5135, -103.3257) -> (-129.8511, -102.6135)
  line L1490 (-129.8511, -102.6135) -> (-130.1629, -101.8908)
  line L1491 (-130.1629, -101.8908) -> (-130.4488, -101.1582)
  line L1492 (-130.4488, -101.1582) -> (-130.7086, -100.4164)
  line L1493 (-130.7086, -100.4164) -> (-130.942, -99.6661)
  line L1494 (-130.942, -99.6661) -> (-131.149, -98.9079)
  line L1495 (-131.149, -98.9079) -> (-131.3292, -98.1425)
  line L1496 (-131.3292, -98.1425) -> (-131.4825, -97.3705)
  line L1497 (-131.4825, -97.3705) -> (-131.6088, -96.5925)
  line L1498 (-131.6088, -96.5925) -> (-131.7078, -95.8094)
  line L1499 (-131.7078, -95.8094) -> (-131.7793, -95.0215)
  line L1500 (-131.7793, -95.0215) -> (-131.8231, -94.2298)
  line L1501 (-131.8231, -94.2298) -> (-131.8392, -93.4347)
  line L1502 (-131.8392, -93.4347) -> (-130.8855, -93.7424)
  line L1503 (-130.8855, -93.7424) -> (-129.9214, -94.0095)
  line L1504 (-129.9214, -94.0095) -> (-128.9476, -94.2358)
  line L1505 (-128.9476, -94.2358) -> (-127.965, -94.4213)
  line L1506 (-127.965, -94.4213) -> (-126.9744, -94.5657)
  line L1507 (-126.9744, -94.5657) -> (-125.9765, -94.6691)
  line L1508 (-125.9765, -94.6691) -> (-124.9722, -94.7312)
  line L1509 (-124.9722, -94.7312) -> (-123.9622, -94.7519)
  line L1510 (-123.9622, -94.7519) -> (-123.3709, -94.7449)
  line L1511 (-123.3709, -94.7449) -> (-122.7817, -94.7237)
  line L1512 (-122.7817, -94.7237) -> (-122.1948, -94.6885)
  line L1513 (-122.1948, -94.6885) -> (-121.6102, -94.6392)
  line L1514 (-121.6102, -94.6392) -> (-121.0282, -94.5758)
  line L1515 (-121.0282, -94.5758) -> (-120.4488, -94.4985)
  line L1516 (-120.4488, -94.4985) -> (-119.8721, -94.4072)
  line L1517 (-119.8721, -94.4072) -> (-119.2984, -94.3019)
  line L1518 (-119.2984, -94.3019) -> (-118.7276, -94.1826)
  line L1519 (-118.7276, -94.1826) -> (-118.16, -94.0495)
  line L1520 (-118.16, -94.0495) -> (-117.5956, -93.9025)
  line L1521 (-117.5956, -93.9025) -> (-117.0346, -93.7416)
  line L1522 (-117.0346, -93.7416) -> (-116.4771, -93.5669)
  line L1523 (-116.4771, -93.5669) -> (-115.9233, -93.3784)
  line L1524 (-115.9233, -93.3784) -> (-115.3732, -93.1761)
  line L1525 (-115.3732, -93.1761) -> (-114.827, -92.9601)
  line L1526 (-114.827, -92.9601) -> (-114.8276, -92.9601)
  line L1527 (-114.8276, -92.9601) -> (-114.6349, -92.8794)
  line L1528 (-114.6349, -92.8794) -> (-113.7817, -92.5022)
  line L1529 (-113.7817, -92.5022) -> (-112.9446, -92.0919)
  line L1530 (-112.9446, -92.0919) -> (-112.1243, -91.6494)
  line L1531 (-112.1243, -91.6494) -> (-111.3219, -91.1756)
  line L1532 (-111.3219, -91.1756) -> (-110.5384, -90.6712)
  line L1533 (-110.5384, -90.6712) -> (-109.7747, -90.1371)
  line L1534 (-109.7747, -90.1371) -> (-109.0318, -89.5742)
  line L1535 (-109.0318, -89.5742) -> (-108.3106, -88.9833)
  line L1536 (-108.3106, -88.9833) -> (-107.6122, -88.3653)
  line L1537 (-107.6122, -88.3653) -> (-106.9375, -87.721)
  line L1538 (-106.9375, -87.721) -> (-106.2874, -87.0513)
  line L1539 (-106.2874, -87.0513) -> (-105.663, -86.357)
  line L1540 (-105.663, -86.357) -> (-105.0652, -85.639)
  line L1541 (-105.0652, -85.639) -> (-104.4949, -84.898)
  line L1542 (-104.4949, -84.898) -> (-103.9532, -84.135)
  line L1543 (-103.9532, -84.135) -> (-103.441, -83.3509)
  line L1544 (-103.441, -83.3509) -> (-103.3468, -84.0947)
  line L1545 (-103.3468, -84.0947) -> (-103.2794, -84.8417)
  line L1546 (-103.2794, -84.8417) -> (-103.2389, -85.5901)
  line L1547 (-103.2389, -85.5901) -> (-103.2254, -86.3383)
  line L1548 (-103.2254, -86.3383) -> (-103.2438, -87.2135)
  line L1549 (-103.2438, -87.2135) -> (-103.2986, -88.0812)
  line L1550 (-103.2986, -88.0812) -> (-103.3891, -88.9405)
  line L1551 (-103.3891, -88.9405) -> (-103.5147, -89.7906)
  line L1552 (-103.5147, -89.7906) -> (-103.6748, -90.6307)
  line L1553 (-103.6748, -90.6307) -> (-103.8686, -91.4598)
  line L1554 (-103.8686, -91.4598) -> (-104.0955, -92.277)
  line L1555 (-104.0955, -92.277) -> (-104.3548, -93.0817)
  line L1556 (-104.3548, -93.0817) -> (-104.6459, -93.8728)
  line L1557 (-104.6459, -93.8728) -> (-104.9682, -94.6496)
  line L1558 (-104.9682, -94.6496) -> (-105.3209, -95.4111)
  line L1559 (-105.3209, -95.4111) -> (-105.7034, -96.1566)
  line L1560 (-105.7034, -96.1566) -> (-106.1151, -96.8851)
  line L1561 (-106.1151, -96.8851) -> (-106.5553, -97.5959)
  line L1562 (-106.5553, -97.5959) -> (-107.0233, -98.288)
  line L1563 (-107.0233, -98.288) -> (-107.5185, -98.9606)
  line L1564 (-107.5185, -98.9606) -> (-108.0403, -99.6128)
  line L1565 (-108.0403, -99.6128) -> (-108.5879, -100.2438)
  line L1566 (-108.5879, -100.2438) -> (-109.1607, -100.8527)
  line L1567 (-109.1607, -100.8527) -> (-109.758, -101.4387)
  line L1568 (-109.758, -101.4387) -> (-110.3793, -102.0009)
  line L1569 (-110.3793, -102.0009) -> (-111.0237, -102.5385)
  line L1570 (-111.0237, -102.5385) -> (-111.6908, -103.0505)
  line L1571 (-111.6908, -103.0505) -> (-112.3798, -103.5362)
  line L1572 (-112.3798, -103.5362) -> (-113.09, -103.9947)
  line L1573 (-113.09, -103.9947) -> (-113.8208, -104.4251)
  line L1574 (-113.8208, -104.4251) -> (-114.5716, -104.8265)
  line L1575 (-114.5716, -104.8265) -> (-115.3417, -105.1982)
  line L1576 (-115.3417, -105.1982) -> (-116.1304, -105.5392)
  line L1577 (-116.1304, -105.5392) -> (-116.937, -105.8487)
  line L1578 (-116.937, -105.8487) -> (-117.761, -106.1259)
  line L1579 (-117.761, -106.1259) -> (-118.6017, -106.3698)
  line L1580 (-118.6017, -106.3698) -> (-118.8432, -106.4349)
  line L1581 (-118.8432, -106.4349) -> (-119.7328, -106.6403)
  line L1582 (-119.7328, -106.6403) -> (-119.9984, -106.6939)
  line L1583 (-119.9984, -106.6939) -> (-120.4868, -106.7827)
  line L1584 (-120.4868, -106.7827) -> (-120.9781, -106.8598)
  line L1585 (-120.9781, -106.8598) -> (-121.4718, -106.9252)
  line L1586 (-121.4718, -106.9252) -> (-121.9676, -106.9788)
  line L1587 (-121.9676, -106.9788) -> (-122.4649, -107.0206)
  line L1588 (-122.4649, -107.0206) -> (-122.9633, -107.0505)
  line L1589 (-122.9633, -107.0505) -> (-123.4624, -107.0685)
  line L1590 (-123.4624, -107.0685) -> (-123.9616, -107.0745)
  line L1591 (-123.9616, -107.0745) -> (-123.9622, -107.0757)
  point P0 (0, 0)
  point P1 (119.3059, -91.2529)
  constraints: 3184 end point
extrude "Extrusion11" cut sketch "Sketch5" against normal through all
fillet "Fillet5" radius 6.35 8 edges at (-139.7, 114.3, 9.525) (-152.4, 127, 1.5875) (0, 114.3, 9.525) (152.4, 127, 1.5875) (-139.7, -38.1, 9.525) (0, -38.1, 9.525) (152.4, -127, 1.5875) (-152.4, -127, 1.5875)
fillet "Fillet1" radius 3.175 9 edges at (-69.85, 101.6, 3.175) (-120.65, 88.9, 3.175) (-69.85, 76.2, 3.175) (-19.05, 88.9, 3.175) (-19.05, 101.6, 9.525) (-120.65, 101.6, 9.525) (-120.65, 76.2, 9.525) (-19.05, 76.2, 9.525) (-63.5, 38.1, 3.175)
fillet "Fillet2" radius 3.175 2 edges at (34.925, 19.05, 9.525) (15.875, 19.05, 9.525)
fillet "Fillet3" radius 1.5875 4 edges at (0, 38.1, 3.175) (-69.85, -38.1, 3.175) (-69.85, 114.3, 3.175) (-139.7, 38.1, 3.175)
fillet "Fillet4" radius 1.5875 12 edges at (76.2, -38.1, 3.175) (19.05, -28.575, 3.175) (133.35, -28.575, 3.175) (131.5169, -36.2669, 6.35) (131.5169, -20.8831, 6.35) (129.6838, -28.575, 9.525) (76.2, -34.4338, 9.525) (76.2, -22.7162, 9.525) (76.2, -19.05, 3.175) (22.7162, -28.575, 9.525) (20.8831, -36.2669, 6.35) (20.8831, -20.8831, 6.35)
body "Solid1"
